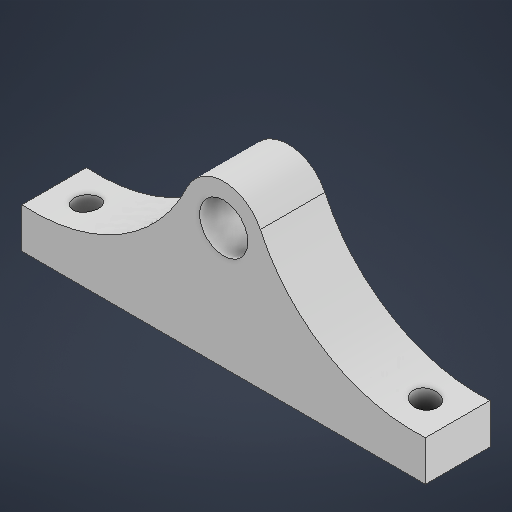
# Autodesk Inventor part: podstawa
Saved by Autodesk Inventor 2026.2 (Build 302298000, 298)
## iProperties
Created: 2025-11-25
Part Number: podstawa
Material: Generic
Document SubType Name: Modeling
Designer: janek
Density: 1 g/cm^3
Appearance: Default
Author: janek
Autodesk Inventor part; units mm, degrees
ref_plane "YZ Plane" through (0, 0, 0) normal (1, 0, 0) x (0, 1, 0)
ref_plane "XZ Plane" through (0, 0, 0) normal (0, 1, 0) x (-1, 0, 0)
ref_plane "XY Plane" through (0, 0, 0) normal (0, 0, 1) x (1, 0, 0)
sketch "Sketch1" plane through (0, 0, 0) normal (0, 0, 1) x (1, 0, 0)
  line L0 (0, 0) -> (50, 0)
  line L1 (50, 0) -> (50, 5)
  line L2 (50, 5) -> (0, 5)
  line L3 (0, 5) -> (0, 0)
  line L4 (20, 5) -> (30, 5)
  line L5 (30, 5) -> (30, 15)
  line L6 (30, 15) -> (20, 15)
  line L7 (20, 15) -> (20, 5)
  circle A0 centre (25, 15) radius 5
  arc A1 (0, 5) -> (20.4903, 17.1592) centre (1.4197, 25.952) ccw
  arc A2 (29.5348, 17.1062) -> (50, 5) centre (48.5808, 25.952) ccw
  circle A3 centre (25, 15) radius 3
  point P0 (50, 2.5)
  point P1 (0, 2.5)
  dimension "d0" = 50
  dimension "d1" = 5
  dimension "d2" = 10
  dimension "d3" = 20
  dimension "d4" = 15
  dimension "d5" = 21
  dimension "d7" = 21
  dimension "d8" = 12.1592
  dimension "d9" = 6
  constraints: 16 end point, 7 point on circle, 4 centre point, 4 parallel, 3 midpoint, 2 horizontal, 2 perpendicular, 1 coincident, 1 point on line, 1 tangent
  measures "d0" distance from line of point (50, 2.5) L3
  measures "d1" distance between parallel lines of L0 L2
  measures "d2" distance of L5.end L6.end
  measures "d3" distance from line of point (0, 2.5) L7
  measures "d4" distance between parallel lines of L0 L6
  measures "d5" radius of A1
  measures "d7" radius of A2
  measures "d8" distance from line of L2 A0.end
  measures "d9" diameter of A3
extrude "Extrusion1" add sketch "Sketch1" along normal blind 8 contours L3 A1 L2 A2 L1 L0 | A0 L6 A3 | A1 A0 L7 L2 | L2 L5 A0 A2 | L7 A0 L5 L2 | L6 A3 A0
sketch "Sketch2" plane through (0, 0, 0) normal (0, -1, 0) x (1, 0, 0)
  line L0 (0, 8) -> (50, 8) projected
  line L1 (0, 0) -> (0, 8) projected
  line L2 (50, 0) -> (50, 8) projected
  point P0 (4, 4)
  point P1 (46, 4)
  point P2 (50, 4)
  dimension "d12" = 4
  dimension "d13" = 4
  dimension "d14" = 4
  dimension "d15" = 4
  constraints: 1 midpoint
  measures "d12" distance from line of L0 point (4, 4)
  measures "d13" distance from line of L1 point (4, 4)
  measures "d14" distance of point (50, 4) point (46, 4)
  measures "d15" distance from line of L0 point (46, 4)
hole "Hole2" at (4, 0, 4) at (46, 0, 4) direction (0, 1, 0) diameter 3 end through all
body "Solid1"
